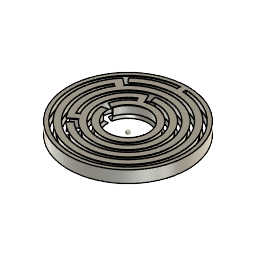
ball-maze v4 (Autodesk Fusion 360 design; units mm, degrees)
Autodesk Fusion 360 part; units mm, degrees
sketch "Sketch1" plane through (0, 0, 0) normal (0, 0, 1) x (1, 0, 0)
  circle A0 centre (0, 0) radius 40
  circle A1 centre (0, 0) radius 39
  circle A2 centre (0, 0) radius 34
  circle A3 centre (0, 0) radius 33
  circle A4 centre (0, 0) radius 28
  circle A5 centre (0, 0) radius 27
  circle A6 centre (0, 0) radius 22
  circle A7 centre (0, 0) radius 21
  circle A8 centre (0, 0) radius 16
  circle A9 centre (0, 0) radius 15
  line L0 (0, 34) -> (0, 39)
  line L1 (-1, 38.9872) -> (-1, 33.9853)
  line L2 (-22.823, 25.2014) -> (-22.1725, 24.4413)
  line L3 (-26.6103, 21.1635) -> (-21.8294, 17.5351)
  line L4 (-26.8651, 19.1643) -> (-22.7932, 16.2625)
  line L5 (-22.4127, -16.783) -> (-17.6772, -13.0964)
  line L6 (-22.5813, -14.8016) -> (-18.463, -11.9631)
  line L7 (-18.3477, -21.151) -> (-17.6483, -20.4337)
  line L8 (-8.8141, 20.1572) -> (-6.2757, 14.7179)
  line L9 (-9.3861, 18.7856) -> (-7.2707, 14.2526)
  line L10 (-3.0247, 21.7911) -> (-2.8086, 20.8113)
  line L11 (-15.2884, 4.7185) -> (-14.3677, 4.3091)
  line L12 (-15.9095, -1.6997) -> (-14.9307, -1.4402)
  dimension "d1" = 80
  dimension "d2" = 78
  dimension "d7" = 68
  dimension "d8" = 66
  dimension "d9" = 56
  dimension "d10" = 54
  dimension "d11" = 44
  dimension "d12" = 42
  dimension "d13" = 32
  dimension "d14" = 30
  dimension "d15" = 1
  constraint coincident A0.centre A1.centre
  constraint concentric A0 A1
  constraint concentric A1 A3
  constraint concentric A0 A4
  constraint concentric A2 A6
  constraint concentric A6 A7
  constraint concentric A1 A8
  constraint concentric A0 A9
  constraint coincident A2 L0.start
  constraint coincident A1 L0.end
  constraint vertical L0
  constraint coincident A1 L1.start
  constraint coincident A2 L1.end
  constraint parallel L0 L1
  constraint coincident A2 L2.start
  constraint coincident A3 L2.end
  constraint coincident A2 L3.start
  constraint coincident A4 L3.end
  constraint coincident A3 L4.start
  constraint coincident A4 L4.end
  constraint coincident A4 L5.start
  constraint coincident A6 L5.end
  constraint coincident A5 L6.start
  constraint coincident A6 L6.end
  constraint coincident A4 L7.start
  constraint coincident A5 L7.end
  constraint coincident A6 L8.start
  constraint coincident A8 L8.end
  constraint coincident A7 L9.start
  constraint coincident A8 L9.end
  constraint parallel L8 L9
  constraint coincident A6 L10.start
  constraint coincident A7 L10.end
  constraint coincident A8 L11.start
  constraint coincident A9 L11.end
  constraint coincident A8 L12.start
  constraint coincident A9 L12.end
  measures "d1" diameter of A0
  measures "d2" diameter of A1
  measures "d7" diameter of A2
  measures "d8" diameter of A3
  measures "d9" diameter of A4
  measures "d10" diameter of A5
  measures "d11" diameter of A6
  measures "d12" diameter of A7
  measures "d13" diameter of A8
  measures "d14" diameter of A9
  measures "d15" distance of L0 L1
extrude "Extrude1" add sketch "Sketch1" along normal blind 5 makes body 1
extrude "Extrude2" add sketch "Sketch1" along normal blind 5 contours A1 A2 L0 L1 picked at (-0.8889, 35.6553) bodies 1
extrude "Extrude3" add sketch "Sketch1" along normal blind 5 contours A2 A3 L2 L3 picked at (-28.5432, 17.1009) bodies 1
extrude "Extrude4" add sketch "Sketch1" along normal blind 5 contours A3 A4 L3 L4 picked at (-24.7148, 19.2587) bodies 1
extrude "Extrude5" add sketch "Sketch1" along normal blind 5 contours A4 A5 L5 L7 picked at (-23.8824, -13.1915) bodies 1
extrude "Extrude6" add sketch "Sketch1" along normal blind 5 contours A5 A6 L5 L6 picked at (-21.0206, -14.1372) bodies 1
extrude "Extrude7" add sketch "Sketch1" along normal blind 5 contours A6 A7 L8 L10 picked at (-19.3498, -8.8935) bodies 1
extrude "Extrude8" add sketch "Sketch1" along normal blind 5 contours A7 A8 L8 L9 picked at (-7.8665, 15.8178) bodies 1
extrude "Extrude9" add sketch "Sketch1" along normal blind 5 contours A8 A9 L11 L12 picked at (-7.1672, 13.5253) bodies 1
sketch "Sketch2" plane through (0, 0, 5) normal (0, 0, 1) x (-1, 0, 0)
  arc A0 (1, -38.9872) -> (0, -39) centre (0, 0) ccw
  line L0 (1, -38.9872) -> (1, -33.9853)
  arc A1 (1, -33.9853) -> (22.823, -25.2014) centre (0, 0) ccw
  line L1 (22.823, -25.2014) -> (22.1725, -24.4413)
  arc A2 (26.8651, -19.1643) -> (22.1725, -24.4413) centre (0, 0) ccw
  line L2 (26.8651, -19.1643) -> (22.7932, -16.2625)
  arc A3 (22.7932, -16.2625) -> (22.4127, 16.783) centre (0, 0) ccw
  line L3 (22.4127, 16.783) -> (17.6772, 13.0964)
  arc A4 (17.6772, 13.0964) -> (3.0247, -21.7911) centre (0, 0) ccw
  line L4 (3.0247, -21.7911) -> (2.8086, -20.8113)
  arc A5 (9.3861, -18.7856) -> (2.8086, -20.8113) centre (0, 0) ccw
  line L5 (9.3861, -18.7856) -> (7.2707, -14.2526)
  arc A6 (7.2707, -14.2526) -> (15.2884, -4.7185) centre (0, 0) ccw
  line L6 (15.2884, -4.7185) -> (14.3677, -4.3091)
  arc A7 (14.9307, 1.4402) -> (14.3677, -4.3091) centre (0, 0) ccw
  line L7 (14.9307, 1.4402) -> (15.9095, 1.6997)
  arc A8 (15.9095, 1.6997) -> (6.2757, -14.7179) centre (0, 0) ccw
  line L8 (6.2757, -14.7179) -> (8.8141, -20.1572)
  arc A9 (8.8141, -20.1572) -> (18.463, 11.9631) centre (0, 0) ccw
  line L9 (18.463, 11.9631) -> (22.5813, 14.8016)
  arc A10 (17.6483, 20.4337) -> (22.5813, 14.8016) centre (0, 0) ccw
  line L10 (17.6483, 20.4337) -> (18.3477, 21.151)
  arc A11 (18.3477, 21.151) -> (21.8294, -17.5351) centre (0, 0) ccw
  line L11 (21.8294, -17.5351) -> (26.6103, -21.1635)
  arc A12 (26.6103, -21.1635) -> (0, -34) centre (0, 0) ccw
  line L12 (0, -34) -> (0, -39)
  circle A13 centre (0, 0) radius 40
  line L13 (17.0672, -3.8677) -> (13.3193, -2.2014)
  arc A14 (13.491, -0.4934) -> (13.3193, -2.2014) centre (0, 0) ccw
  line L14 (13.491, -0.4934) -> (17.4908, 0.5672)
  arc A15 (17.4908, 0.5672) -> (5.5043, -16.6118) centre (0, 0) ccw
  line L15 (5.5043, -16.6118) -> (8.0545, -22.0766)
  arc A16 (8.0545, -22.0766) -> (20.4773, 11.5296) centre (0, 0) ccw
  line L16 (20.4773, 11.5296) -> (22.1303, 12.6689)
  arc A17 (17.7093, 18.3475) -> (22.1303, 12.6689) centre (0, 0) ccw
  line L17 (17.7093, 18.3475) -> (20.5017, 21.2116)
  arc A18 (20.5017, 21.2116) -> (22.0561, -19.5903) centre (0, 0) ccw
  line L18 (22.0561, -19.5903) -> (26.8473, -23.2265)
  arc A19 (26.8473, -23.2265) -> (-1.5, -35.4683) centre (0, 0) ccw
  line L19 (-1.5, -35.4683) -> (-1.5, -37.47)
  arc A20 (2.5, -37.4166) -> (-1.5, -37.47) centre (0, 0) ccw
  line L20 (2.5, -37.4166) -> (2.5, -35.4119)
  arc A21 (2.5, -35.4119) -> (24.8915, -25.3113) centre (0, 0) ccw
  line L21 (24.8915, -25.3113) -> (22.2836, -22.2642)
  arc A22 (26.4855, -17.0519) -> (22.2836, -22.2642) centre (0, 0) ccw
  line L22 (26.4855, -17.0519) -> (24.8549, -15.8898)
  arc A23 (24.8549, -15.8898) -> (22.6661, 18.8812) centre (0, 0) ccw
  line L23 (22.6661, 18.8812) -> (17.9284, 15.1929)
  arc A24 (17.9284, 15.1929) -> (4.8271, -22.9989) centre (0, 0) ccw
  line L24 (4.8271, -22.9989) -> (3.9655, -19.0925)
  arc A25 (10.0681, -16.6998) -> (3.9655, -19.0925) centre (0, 0) ccw
  line L25 (10.0681, -16.6998) -> (9.217, -14.8761)
  arc A26 (9.217, -14.8761) -> (17.0672, -3.8677) centre (0, 0) ccw
  dimension "d35" = -1.5
extrude "Extrude10" add sketch "Sketch2" along normal blind 1.5 contours A0 L0 A1 L1 A2 L2 A3 L3 A4 L4 A5 L5 A6 L6 A7 L7 A8 L8 A9 L9 A10 L10 A11 L11 A12 L12 | A13 bodies 1
chamfer "Chamfer1" distance 1.4 angle 45 25 edges at (13.4323, -1.3501, 5) (-15.1933, 3.0346, 5) (-14.2482, 10.1607, 5) (-9.6425, 15.7879, 5) (7.1181, -18.1544, 5) (-4.3963, 21.0457, 5) (22.2285, -7.6252, 5) (14.3518, -10.0138, 5) (-6.7794, 19.3442, 5) (-22.0422, 8.1481, 5) (-21.3038, -12.0993, 5) (20.1211, 15.665, 5) (-20.2972, -17.037, 5) (-19.1055, -19.7795, 5) (29.4786, 1.123, 5) (-29.4417, -1.8533, 5) (-24.4517, 21.4084, 5) (-25.6702, 16.4708, 5) (14.0743, -32.5908, 5) (-23.5875, 23.7877, 5) (24.5234, -19.77, 5) (1.5, 36.4691, 5) (0.5007, -37.4967, 5) (-2.5, 36.4142, 5) (-14.5972, 32.36, 5) on bodies 1
chamfer "Chamfer2" distance 1.4 angle 45 1 edges at (-15.4991, -0.0391, 5) on bodies 1
sketch "Sketch3" plane through (0, 0, 0) normal (0, 0, -1) x (1, 0, 0)
  arc A0 (0, -39) -> (-1, -38.9872) centre (0, 0) ccw
  line L0 (0, -39) -> (0, -34)
  arc A1 (0, -34) -> (-26.6103, -21.1635) centre (0, 0) ccw
  line L1 (-26.6103, -21.1635) -> (-21.8294, -17.5351)
  arc A2 (-21.8294, -17.5351) -> (-18.3477, 21.151) centre (0, 0) ccw
  line L2 (-18.3477, 21.151) -> (-17.6483, 20.4337)
  arc A3 (-22.5813, 14.8016) -> (-17.6483, 20.4337) centre (0, 0) ccw
  line L3 (-22.5813, 14.8016) -> (-18.463, 11.9631)
  arc A4 (-18.463, 11.9631) -> (-8.8141, -20.1572) centre (0, 0) ccw
  line L4 (-8.8141, -20.1572) -> (-6.2757, -14.7179)
  arc A5 (-6.2757, -14.7179) -> (-15.9095, 1.6997) centre (0, 0) ccw
  line L5 (-15.9095, 1.6997) -> (-14.9307, 1.4402)
  arc A6 (-14.3677, -4.3091) -> (-14.9307, 1.4402) centre (0, 0) ccw
  line L6 (-14.3677, -4.3091) -> (-15.2884, -4.7185)
  arc A7 (-15.2884, -4.7185) -> (-7.2707, -14.2526) centre (0, 0) ccw
  line L7 (-7.2707, -14.2526) -> (-9.3861, -18.7856)
  arc A8 (-2.8086, -20.8113) -> (-9.3861, -18.7856) centre (0, 0) ccw
  line L8 (-2.8086, -20.8113) -> (-3.0247, -21.7911)
  arc A9 (-3.0247, -21.7911) -> (-17.6772, 13.0964) centre (0, 0) ccw
  line L9 (-17.6772, 13.0964) -> (-22.4127, 16.783)
  arc A10 (-22.4127, 16.783) -> (-22.7932, -16.2625) centre (0, 0) ccw
  line L10 (-22.7932, -16.2625) -> (-26.8651, -19.1643)
  arc A11 (-22.1725, -24.4413) -> (-26.8651, -19.1643) centre (0, 0) ccw
  line L11 (-22.1725, -24.4413) -> (-22.823, -25.2014)
  arc A12 (-22.823, -25.2014) -> (-1, -33.9853) centre (0, 0) ccw
  line L12 (-1, -33.9853) -> (-1, -38.9872)
  circle A13 centre (0, 0) radius 40
  line L13 (-2.5, -35.4119) -> (-2.5, -37.4166)
  arc A14 (1.5, -37.47) -> (-2.5, -37.4166) centre (0, 0) ccw
  line L14 (1.5, -37.47) -> (1.5, -35.4683)
  arc A15 (1.5, -35.4683) -> (-26.8473, -23.2265) centre (0, 0) ccw
  line L15 (-26.8473, -23.2265) -> (-22.0561, -19.5903)
  arc A16 (-22.0561, -19.5903) -> (-20.5017, 21.2116) centre (0, 0) ccw
  line L16 (-20.5017, 21.2116) -> (-17.7093, 18.3475)
  arc A17 (-22.1303, 12.6689) -> (-17.7093, 18.3475) centre (0, 0) ccw
  line L17 (-22.1303, 12.6689) -> (-20.4773, 11.5296)
  arc A18 (-20.4773, 11.5296) -> (-8.0545, -22.0766) centre (0, 0) ccw
  line L18 (-8.0545, -22.0766) -> (-5.5043, -16.6118)
  arc A19 (-5.5043, -16.6118) -> (-17.4908, 0.5672) centre (0, 0) ccw
  line L19 (-17.4908, 0.5672) -> (-13.491, -0.4934)
  arc A20 (-13.3193, -2.2014) -> (-13.491, -0.4934) centre (0, 0) ccw
  line L20 (-13.3193, -2.2014) -> (-17.0672, -3.8677)
  arc A21 (-17.0672, -3.8677) -> (-9.217, -14.8761) centre (0, 0) ccw
  line L21 (-9.217, -14.8761) -> (-10.0681, -16.6998)
  arc A22 (-3.9655, -19.0925) -> (-10.0681, -16.6998) centre (0, 0) ccw
  line L22 (-3.9655, -19.0925) -> (-4.8271, -22.9989)
  arc A23 (-4.8271, -22.9989) -> (-17.9284, 15.1929) centre (0, 0) ccw
  line L23 (-17.9284, 15.1929) -> (-22.6661, 18.8812)
  arc A24 (-22.6661, 18.8812) -> (-24.8549, -15.8898) centre (0, 0) ccw
  line L24 (-24.8549, -15.8898) -> (-26.4855, -17.0519)
  arc A25 (-22.2836, -22.2642) -> (-26.4855, -17.0519) centre (0, 0) ccw
  line L25 (-22.2836, -22.2642) -> (-24.8915, -25.3113)
  arc A26 (-24.8915, -25.3113) -> (-2.5, -35.4119) centre (0, 0) ccw
  dimension "d40" = -1.5
extrude "Extrude11" add sketch "Sketch3" along normal blind 1.5 contours A0 L0 A1 L1 A2 L2 A3 L3 A4 L4 A5 L5 A6 L6 A7 L7 A8 L8 A9 L9 A10 L10 A11 L11 A12 L12 | A13 bodies 1
chamfer "Chamfer3" distance 1.4 angle 45 26 edges at (13.4323, -1.3501, 0) (-15.1933, 3.0346, 0) (-15.4909, -0.0369, 0) (-14.2482, 10.1607, 0) (-9.6425, 15.7879, 0) (7.1181, -18.1544, 0) (14.3518, -10.0138, 0) (-6.7794, 19.3442, 0) (-22.0422, 8.1481, 0) (22.2285, -7.6252, 0) (-4.3963, 21.0457, 0) (-21.3038, -12.0993, 0) (20.1211, 15.665, 0) (-19.1055, -19.7795, 0) (-20.2972, -17.037, 0) (-29.4417, -1.8533, 0) (24.5234, -19.77, 0) (-25.6702, 16.4708, 0) (29.4786, 1.123, 0) (-24.4517, 21.4084, 0) (-14.5972, 32.36, 0) (-23.5875, 23.7877, 0) (-2.5, 36.4142, 0) (0.5007, -37.4967, 0) (14.0743, -32.5908, 0) (1.5, 36.4691, 0) on bodies 1
sphere "SpherePrimitive1" add diameter 3 placed x (1, 0, 0) y (0, 1, 0) z (0, 0, 1) at (0, 0, 0) separate body makes body 2
